Autodesk Inventor part; units mm, degrees
(part 2 of 10)
  spline S9 degree 5 poles (-7.9935, -0.3229) (-7.988, -0.3264) (-7.9807, -0.331) (-7.9716, -0.3367) (-7.9607, -0.3435) (-7.948, -0.3514) (-7.9389, -0.357) (-7.9299, -0.3625) (-7.9208, -0.368) (-7.9118, -0.3735) (-7.9028, -0.3789) (-7.8937, -0.3843) (-7.8847, -0.3897) (-7.8757, -0.3951) (-7.8667, -0.4004) (-7.8578, -0.4056) (-7.8488, -0.4109) (-7.8398, -0.4161) (-7.8309, -0.4212) (-7.822, -0.4263) (-7.813, -0.4314) (-7.8041, -0.4365) (-7.7952, -0.4415) (-7.7863, -0.4465) (-7.7775, -0.4514) (-7.7686, -0.4563) (-7.7598, -0.4612) (-7.7509, -0.4661) (-7.7421, -0.4709) (-7.7333, -0.4756) (-7.7227, -0.4813) (-7.7122, -0.487) (-7.7017, -0.4925) (-7.6912, -0.4981) (-7.6772, -0.5054) (-7.665, -0.5117) (-7.6529, -0.5179) (-7.6408, -0.5241) (-7.6252, -0.5319) (-7.6131, -0.538) (-7.6011, -0.5439) (-7.5891, -0.5498) (-7.5737, -0.5573) (-7.5618, -0.563) (-7.5499, -0.5687) (-7.5364, -0.5751) (-7.5229, -0.5814) (-7.5128, -0.586) (-7.501, -0.5914) (-7.4893, -0.5967) (-7.4793, -0.6013) (-7.4677, -0.6065) (-7.4561, -0.6116) (-7.4462, -0.6159) (-7.4346, -0.6209) (-7.4231, -0.6259) (-7.4133, -0.6301) (-7.4019, -0.6349) (-7.3905, -0.6397) (-7.3808, -0.6437) (-7.3695, -0.6483) (-7.3582, -0.6529) (-7.3486, -0.6568) (-7.3374, -0.6612) (-7.3263, -0.6656) (-7.3168, -0.6693) (-7.3057, -0.6736) (-7.2947, -0.6778) (-7.2853, -0.6814) (-7.2744, -0.6855) (-7.2635, -0.6895) (-7.2542, -0.6929) (-7.2434, -0.6968) (-7.2327, -0.7006) (-7.2235, -0.7039) (-7.2129, -0.7076) (-7.2023, -0.7113) (-7.1932, -0.7144) (-7.1827, -0.718) (-7.1723, -0.7215) (-7.1634, -0.7244) (-7.153, -0.7278) (-7.1427, -0.7311) (-7.134, -0.7339) (-7.1238, -0.7371) (-7.1136, -0.7403) (-7.105, -0.7429) (-7.095, -0.746) (-7.085, -0.749) (-7.0765, -0.7515) (-7.0666, -0.7544) (-7.0568, -0.7572) (-7.0485, -0.7595) (-7.0388, -0.7623) (-7.0292, -0.7649) (-7.021, -0.7671) (-7.0114, -0.7697) (-7.002, -0.7722) (-6.9939, -0.7743) (-6.9846, -0.7767) (-6.9754, -0.779) (-6.9675, -0.781) (-6.9583, -0.7832) (-6.9493, -0.7854) (-6.9416, -0.7872) (-6.9326, -0.7893) (-6.9237, -0.7913) (-6.9162, -0.793) (-6.9075, -0.7949) (-6.8988, -0.7968) (-6.8914, -0.7984) (-6.8829, -0.8002) (-6.8744, -0.8019) (-6.8673, -0.8033) (-6.8589, -0.805) (-6.8507, -0.8066) (-6.8437, -0.8079) (-6.8356, -0.8094) (-6.8276, -0.8108) (-6.8208, -0.812) (-6.8129, -0.8134) (-6.8052, -0.8147) (-6.7986, -0.8158) (-6.7909, -0.8171) (-6.7834, -0.8182) (-6.777, -0.8192) (-6.7696, -0.8203) (-6.7623, -0.8214) (-6.7561, -0.8223) (-6.749, -0.8232) (-6.7419, -0.8242) (-6.736, -0.8249) (-6.7291, -0.8258) (-6.7223, -0.8266) (-6.7166, -0.8273) (-6.7099, -0.828) (-6.7034, -0.8287) (-6.6979, -0.8293) (-6.6916, -0.83) (-6.6853, -0.8306) (-6.6801, -0.8311) (-6.674, -0.8316) (-6.668, -0.8321) (-6.663, -0.8325) (-6.6573, -0.8329) (-6.6516, -0.8333) (-6.6468, -0.8337) (-6.6406, -0.8341) (-6.6345, -0.8344) (-6.6292, -0.8347) (-6.6241, -0.8349) (-6.617, -0.8353) (-6.6115, -0.8355) (-6.6061, -0.8356) (-6.6009, -0.8358) (-6.5959, -0.8359) (-6.5922, -0.836) (-6.5885, -0.836) (-6.585, -0.836) (-6.5816, -0.8361) (-6.5782, -0.8361) (-6.5755, -0.8361) (-6.5729, -0.8361) (-6.5703, -0.836) (-6.5678, -0.836) (-6.5653, -0.836) (-6.5629, -0.8359) (-6.5606, -0.8359) (-6.5583, -0.8358) (-6.5561, -0.8358) (-6.554, -0.8357) (-6.5519, -0.8356) (-6.55, -0.8356) (-6.548, -0.8355) (-6.5462, -0.8354) (-6.5444, -0.8353) (-6.5427, -0.8352) (-6.5411, -0.8351) (-6.5395, -0.835) (-6.5381, -0.8349) (-6.5366, -0.8349) (-6.5353, -0.8348) (-6.5341, -0.8347) (-6.5329, -0.8346) (-6.5318, -0.8345) (-6.5307, -0.8344) (-6.5298, -0.8343) (-6.5289, -0.8343) (-6.5281, -0.8342) (-6.5274, -0.8341) (-6.5267, -0.834) (-6.5262, -0.834) (-6.5258, -0.8339) (-6.5256, -0.8339) (-6.5254, -0.8339) knots -1 -1 -1 -1 -1 -1 -0.9875 -0.983333 -0.979167 -0.975 -0.970833 -0.966667 -0.9625 -0.958333 -0.954167 -0.95 -0.945833 -0.941667 -0.9375 -0.933333 -0.929167 -0.925 -0.920833 -0.916667 -0.9125 -0.908333 -0.904167 -0.9 -0.895833 -0.891667 -0.8875 -0.883333 -0.879167 -0.875 -0.870833 -0.8625 -0.858333 -0.854167 -0.85 -0.8375 -0.833333 -0.829167 -0.825 -0.8125 -0.808333 -0.804167 -0.8 -0.7875 -0.783333 -0.779167 -0.770833 -0.766667 -0.7625 -0.754167 -0.75 -0.745833 -0.7375 -0.733333 -0.729167 -0.720833 -0.716667 -0.7125 -0.704167 -0.7 -0.695833 -0.6875 -0.683333 -0.679167 -0.670833 -0.666667 -0.6625 -0.654167 -0.65 -0.645833 -0.6375 -0.633333 -0.629167 -0.620833 -0.616667 -0.6125 -0.604167 -0.6 -0.595833 -0.5875 -0.583333 -0.579167 -0.570833 -0.566667 -0.5625 -0.554167 -0.55 -0.545833 -0.5375 -0.533333 -0.529167 -0.520833 -0.516667 -0.5125 -0.504167 -0.5 -0.495833 -0.4875 -0.483333 -0.479167 -0.470833 -0.466667 -0.4625 -0.454167 -0.45 -0.445833 -0.4375 -0.433333 -0.429167 -0.420833 -0.416667 -0.4125 -0.404167 -0.4 -0.395833 -0.3875 -0.383333 -0.379167 -0.370833 -0.366667 -0.3625 -0.354167 -0.35 -0.345833 -0.3375 -0.333333 -0.329167 -0.320833 -0.316667 -0.3125 -0.304167 -0.3 -0.295833 -0.2875 -0.283333 -0.279167 -0.270833 -0.266667 -0.2625 -0.254167 -0.25 -0.245833 -0.2375 -0.233333 -0.229167 -0.220833 -0.216667 -0.2125 -0.2 -0.195833 -0.191667 -0.1875 -0.170833 -0.166667 -0.1625 -0.158333 -0.154167 -0.145833 -0.141667 -0.1375 -0.133333 -0.129167 -0.125 -0.120833 -0.116667 -0.1125 -0.108333 -0.104167 -0.1 -0.095833 -0.091667 -0.0875 -0.083333 -0.079167 -0.075 -0.070833 -0.066667 -0.0625 -0.058333 -0.054167 -0.05 -0.045833 -0.041667 -0.0375 -0.033333 -0.029167 -0.025 -0.020833 -0.016667 -0.0125 -0.008333 0 0 0 0 0 0
  line L19 (-6.2404, 2.0798) -> (-5.455, 1.818)
  spline S10 degree 5 poles (-1.4639, -7.8649) (-1.4593, -7.8604) (-1.4532, -7.8543) (-1.4456, -7.8467) (-1.4365, -7.8376) (-1.426, -7.8269) (-1.4186, -7.8193) (-1.4111, -7.8117) (-1.4038, -7.8041) (-1.3964, -7.7965) (-1.3891, -7.7889) (-1.3818, -7.7813) (-1.3746, -7.7738) (-1.3674, -7.7662) (-1.3602, -7.7586) (-1.3531, -7.751) (-1.346, -7.7434) (-1.3389, -7.7359) (-1.3319, -7.7283) (-1.3249, -7.7207) (-1.318, -7.7132) (-1.311, -7.7056) (-1.3042, -7.698) (-1.2973, -7.6905) (-1.2905, -7.6829) (-1.2838, -7.6754) (-1.2771, -7.6678) (-1.2704, -7.6603) (-1.2637, -7.6528) (-1.2571, -7.6452) (-1.2492, -7.6362) (-1.2414, -7.6272) (-1.2336, -7.6182) (-1.2259, -7.6092) (-1.2156, -7.5972) (-1.2068, -7.5867) (-1.198, -7.5763) (-1.1893, -7.5658) (-1.1782, -7.5524) (-1.1696, -7.542) (-1.1611, -7.5316) (-1.1527, -7.5212) (-1.142, -7.5079) (-1.1338, -7.4975) (-1.1256, -7.4872) (-1.1163, -7.4754) (-1.1072, -7.4636) (-1.1004, -7.4548) (-1.0925, -7.4446) (-1.0847, -7.4343) (-1.0781, -7.4256) (-1.0705, -7.4154) (-1.0629, -7.4052) (-1.0564, -7.3965) (-1.049, -7.3864) (-1.0416, -7.3763) (-1.0353, -7.3676) (-1.0281, -7.3576) (-1.0209, -7.3475) (-1.0148, -7.339) (-1.0078, -7.329) (-1.0008, -7.319) (-0.9949, -7.3105) (-0.9881, -7.3006) (-0.9813, -7.2907) (-0.9756, -7.2823) (-0.969, -7.2724) (-0.9624, -7.2626) (-0.9569, -7.2543) (-0.9504, -7.2445) (-0.9441, -7.2348) (-0.9387, -7.2265) (-0.9325, -7.2169) (-0.9263, -7.2073) (-0.9211, -7.199) (-0.9151, -7.1895) (-0.9092, -7.18) (-0.9042, -7.1719) (-0.8984, -7.1624) (-0.8926, -7.153) (-0.8878, -7.145) (-0.8822, -7.1356) (-0.8766, -7.1263) (-0.8719, -7.1184) (-0.8665, -7.1092) (-0.8612, -7.1) (-0.8567, -7.0922) (-0.8515, -7.0831) (-0.8464, -7.074) (-0.842, -7.0663) (-0.837, -7.0573) (-0.8321, -7.0484) (-0.8279, -7.0408) (-0.8231, -7.0319) (-0.8184, -7.0231) (-0.8144, -7.0156) (-0.8098, -7.0069) (-0.8053, -6.9983) (-0.8014, -6.9909) (-0.797, -6.9823) (-0.7927, -6.9738) (-0.789, -6.9666) (-0.7842, -6.957) (-0.7795, -6.9474) (-0.7754, -6.9391) (-0.7715, -6.9309) (-0.7664, -6.9204) (-0.7626, -6.9123) (-0.7588, -6.9043) (-0.7551, -6.8963) (-0.7499, -6.885) (-0.7459, -6.876) (-0.7419, -6.8672) (-0.7381, -6.8584) (-0.7334, -6.8476) (-0.7301, -6.84) (-0.727, -6.8326) (-0.7239, -6.8252) (-0.7196, -6.8148) (-0.7162, -6.8065) (-0.7129, -6.7984) (-0.7097, -6.7903) (-0.7059, -6.7804) (-0.7032, -6.7736) (-0.7006, -6.7668) (-0.6981, -6.7601) (-0.695, -6.7516) (-0.6926, -6.745) (-0.6903, -6.7386) (-0.6877, -6.7313) (-0.6852, -6.7242) (-0.6834, -6.7189) (-0.6813, -6.7128) (-0.6793, -6.7068) (-0.6776, -6.7017) (-0.6757, -6.6958) (-0.6738, -6.6901) (-0.6723, -6.6852) (-0.6705, -6.6796) (-0.6689, -6.6741) (-0.6674, -6.6695) (-0.6658, -6.6642) (-0.6643, -6.6589) (-0.663, -6.6545) (-0.6614, -6.6488) (-0.6598, -6.6432) (-0.6585, -6.6383) (-0.6572, -6.6336) (-0.656, -6.6291) (-0.6548, -6.6245) (-0.6537, -6.6201) (-0.6526, -6.6159) (-0.6516, -6.6117) (-0.6506, -6.6077) (-0.65, -6.6048) (-0.6493, -6.6021) (-0.6487, -6.5994) (-0.6481, -6.5967) (-0.6475, -6.5941) (-0.6469, -6.5916) (-0.6464, -6.5891) (-0.6459, -6.5867) (-0.6454, -6.5844) (-0.6449, -6.5821) (-0.6445, -6.5799) (-0.6441, -6.5777) (-0.6437, -6.5756) (-0.6433, -6.5736) (-0.6429, -6.5717) (-0.6425, -6.5698) (-0.6422, -6.568) (-0.6419, -6.5662) (-0.6416, -6.5645) (-0.6413, -6.5629) (-0.6411, -6.5614) (-0.6408, -6.5599) (-0.6406, -6.5585) (-0.6404, -6.5572) (-0.6402, -6.556) (-0.64, -6.5548) (-0.6399, -6.5537) (-0.6397, -6.5527) (-0.6396, -6.5517) (-0.6395, -6.5509) (-0.6394, -6.5501) (-0.6393, -6.5494) (-0.6392, -6.5486) (-0.6391, -6.5481) (-0.6391, -6.5478) (-0.6391, -6.5475) (-0.6391, -6.5474) knots -1 -1 -1 -1 -1 -1 -0.9875 -0.983333 -0.979167 -0.975 -0.970833 -0.966667 -0.9625 -0.958333 -0.954167 -0.95 -0.945833 -0.941667 -0.9375 -0.933333 -0.929167 -0.925 -0.920833 -0.916667 -0.9125 -0.908333 -0.904167 -0.9 -0.895833 -0.891667 -0.8875 -0.883333 -0.879167 -0.875 -0.870833 -0.8625 -0.858333 -0.854167 -0.85 -0.8375 -0.833333 -0.829167 -0.825 -0.8125 -0.808333 -0.804167 -0.8 -0.7875 -0.783333 -0.779167 -0.770833 -0.766667 -0.7625 -0.754167 -0.75 -0.745833 -0.7375 -0.733333 -0.729167 -0.720833 -0.716667 -0.7125 -0.704167 -0.7 -0.695833 -0.6875 -0.683333 -0.679167 -0.670833 -0.666667 -0.6625 -0.654167 -0.65 -0.645833 -0.6375 -0.633333 -0.629167 -0.620833 -0.616667 -0.6125 -0.604167 -0.6 -0.595833 -0.5875 -0.583333 -0.579167 -0.570833 -0.566667 -0.5625 -0.554167 -0.55 -0.545833 -0.5375 -0.533333 -0.529167 -0.520833 -0.516667 -0.5125 -0.504167 -0.5 -0.495833 -0.4875 -0.483333 -0.479167 -0.470833 -0.466667 -0.4625 -0.45 -0.445833 -0.441667 -0.4375 -0.425 -0.420833 -0.416667 -0.4125 -0.395833 -0.391667 -0.3875 -0.383333 -0.370833 -0.366667 -0.3625 -0.358333 -0.341667 -0.3375 -0.333333 -0.329167 -0.316667 -0.3125 -0.308333 -0.304167 -0.291667 -0.2875 -0.283333 -0.275 -0.270833 -0.266667 -0.258333 -0.254167 -0.25 -0.241667 -0.2375 -0.233333 -0.225 -0.220833 -0.216667 -0.208333 -0.204167 -0.2 -0.1875 -0.183333 -0.179167 -0.175 -0.170833 -0.158333 -0.154167 -0.15 -0.145833 -0.141667 -0.1375 -0.133333 -0.129167 -0.125 -0.120833 -0.116667 -0.1125 -0.108333 -0.104167 -0.1 -0.095833 -0.091667 -0.0875 -0.083333 -0.079167 -0.075 -0.070833 -0.066667 -0.0625 -0.058333 -0.054167 -0.05 -0.045833 -0.041667 -0.0375 -0.033333 -0.029167 -0.025 -0.020833 -0.016667 -0.0125 -0.008333 0 0 0 0 0 0
  line L20 (-1.9798, -5.3984) -> (-2.2648, -6.1757)
  line L21 (-2.2648, -6.1757) -> (-2.265, -6.1763)
  arc A11 (-2.9863, -4.9137) -> (-1.9798, -5.3984) centre (0, 0) ccw
  spline S11 degree 5 poles (-2.265, -6.1763) (-2.2651, -6.1763) (-2.2651, -6.1765) (-2.2652, -6.1767) (-2.2653, -6.177) (-2.2655, -6.1776) (-2.2657, -6.1782) (-2.2659, -6.1788) (-2.2662, -6.1796) (-2.2664, -6.1804) (-2.2667, -6.1813) (-2.267, -6.1823) (-2.2674, -6.1834) (-2.2677, -6.1845) (-2.2681, -6.1857) (-2.2685, -6.187) (-2.2689, -6.1883) (-2.2693, -6.1898) (-2.2697, -6.1913) (-2.2702, -6.1928) (-2.2706, -6.1945) (-2.2711, -6.1962) (-2.2716, -6.198) (-2.2721, -6.1998) (-2.2726, -6.2017) (-2.2732, -6.2037) (-2.2737, -6.2058) (-2.2742, -6.2079) (-2.2748, -6.2101) (-2.2754, -6.2123) (-2.2759, -6.2147) (-2.2765, -6.2171) (-2.2771, -6.2195) (-2.2777, -6.222) (-2.2783, -6.2246) (-2.279, -6.2278) (-2.2798, -6.2311) (-2.2805, -6.2344) (-2.2815, -6.2391) (-2.2828, -6.2451) (-2.2839, -6.2507) (-2.2851, -6.2565) (-2.2862, -6.2625) (-2.2875, -6.2694) (-2.2885, -6.2751) (-2.2895, -6.281) (-2.2906, -6.287) (-2.2918, -6.2947) (-2.2927, -6.3002) (-2.2935, -6.3058) (-2.2944, -6.3115) (-2.2956, -6.3199) (-2.2966, -6.3268) (-2.2975, -6.3338) (-2.2984, -6.3409) (-2.2995, -6.35) (-2.3003, -6.3565) (-2.301, -6.3631) (-2.3017, -6.3698) (-2.3027, -6.3786) (-2.3033, -6.3855) (-2.304, -6.3925) (-2.3047, -6.4007) (-2.3055, -6.4089) (-2.306, -6.4152) (-2.3065, -6.4216) (-2.3072, -6.4312) (-2.3078, -6.4399) (-2.3083, -6.4488) (-2.3089, -6.4577) (-2.3095, -6.4691) (-2.3099, -6.4771) (-2.3102, -6.4853) (-2.3106, -6.4935) (-2.3109, -6.5042) (-2.3112, -6.5127) (-2.3114, -6.5212) (-2.3116, -6.5298) (-2.3119, -6.5422) (-2.312, -6.5523) (-2.3121, -6.5625) (-2.3121, -6.5728) (-2.3121, -6.5858) (-2.3121, -6.595) (-2.312, -6.6043) (-2.3119, -6.6136) (-2.3117, -6.6258) (-2.3115, -6.6353) (-2.3112, -6.6449) (-2.3109, -6.656) (-2.3105, -6.6672) (-2.3102, -6.6756) (-2.3097, -6.6856) (-2.3093, -6.6956) (-2.3089, -6.7042) (-2.3083, -6.7143) (-2.3077, -6.7245) (-2.3072, -6.7333) (-2.3065, -6.7437) (-2.3058, -6.7541) (-2.3052, -6.763) (-2.3044, -6.7736) (-2.3036, -6.7842) (-2.3028, -6.7933) (-2.3019, -6.804) (-2.301, -6.8148) (-2.3001, -6.8241) (-2.299, -6.8351) (-2.2979, -6.846) (-2.297, -6.8555) (-2.2958, -6.8666) (-2.2945, -6.8778) (-2.2934, -6.8874) (-2.2921, -6.8987) (-2.2907, -6.91) (-2.2895, -6.9198) (-2.288, -6.9312) (-2.2865, -6.9428) (-2.2852, -6.9527) (-2.2836, -6.9643) (-2.2819, -6.976) (-2.2804, -6.9861) (-2.2787, -6.9979) (-2.2768, -7.0097) (-2.2752, -7.0199) (-2.2733, -7.0319) (-2.2714, -7.0439) (-2.2696, -7.0542) (-2.2676, -7.0663) (-2.2654, -7.0785) (-2.2636, -7.089) (-2.2614, -7.1012) (-2.2591, -7.1136) (-2.2571, -7.1242) (-2.2547, -7.1366) (-2.2523, -7.1491) (-2.2501, -7.1598) (-2.2476, -7.1724) (-2.245, -7.185) (-2.2427, -7.1958) (-2.24, -7.2085) (-2.2372, -7.2213) (-2.2348, -7.2323) (-2.2324, -7.2433) (-2.2295, -7.2562) (-2.2269, -7.2672) (-2.2243, -7.2784) (-2.2212, -7.2914) (-2.2177, -7.3063) (-2.2145, -7.3194) (-2.2112, -7.3326) (-2.2074, -7.3476) (-2.2035, -7.3628) (-2.2001, -7.3761) (-2.196, -7.3913) (-2.1919, -7.4066) (-2.1883, -7.4201) (-2.1851, -7.4316) (-2.1818, -7.4432) (-2.1791, -7.4529) (-2.1764, -7.4626) (-2.1736, -7.4723) (-2.1708, -7.482) (-2.1679, -7.4918) (-2.165, -7.5015) (-2.1621, -7.5113) (-2.1592, -7.5211) (-2.1562, -7.531) (-2.1532, -7.5408) (-2.1501, -7.5507) (-2.1471, -7.5606) (-2.144, -7.5705) (-2.1408, -7.5804) (-2.1377, -7.5904) (-2.1345, -7.6003) (-2.1312, -7.6103) (-2.128, -7.6203) (-2.1247, -7.6303) (-2.1213, -7.6403) (-2.118, -7.6504) (-2.1146, -7.6605) (-2.1091, -7.6766) (-2.1042, -7.6907) (-2.1, -7.7029) (-2.0964, -7.7131) (-2.0935, -7.7212) knots 0 0 0 0 0 0 0.004167 0.008333 0.0125 0.016667 0.020833 0.025 0.029167 0.033333 0.0375 0.041667 0.045833 0.05 0.054167 0.058333 0.0625 0.066667 0.070833 0.075 0.079167 0.083333 0.0875 0.091667 0.095833 0.1 0.104167 0.108333 0.1125 0.116667 0.120833 0.125 0.129167 0.133333 0.1375 0.141667 0.15 0.154167 0.158333 0.170833 0.183333 0.1875 0.191667 0.195833 0.2125 0.216667 0.220833 0.225 0.2375 0.241667 0.245833 0.25 0.266667 0.270833 0.275 0.279167 0.291667 0.295833 0.3 0.304167 0.316667 0.320833 0.325 0.333333 0.3375 0.341667 0.345833 0.3625 0.366667 0.370833 0.375 0.3875 0.391667 0.395833 0.4 0.4125 0.416667 0.420833 0.425 0.441667 0.445833 0.45 0.454167 0.466667 0.470833 0.475 0.479167 0.491667 0.495833 0.5 0.508333 0.5125 0.516667 0.525 0.529167 0.533333 0.541667 0.545833 0.55 0.558333 0.5625 0.566667 0.575 0.579167 0.583333 0.591667 0.595833 0.6 0.608333 0.6125 0.616667 0.625 0.629167 0.633333 0.641667 0.645833 0.65 0.658333 0.6625 0.666667 0.675 0.679167 0.683333 0.691667 0.695833 0.7 0.708333 0.7125 0.716667 0.725 0.729167 0.733333 0.741667 0.745833 0.75 0.758333 0.7625 0.766667 0.775 0.779167 0.783333 0.791667 0.795833 0.8 0.804167 0.8125 0.816667 0.820833 0.829167 0.8375 0.841667 0.845833 0.854167 0.8625 0.866667 0.875 0.879167 0.883333 0.8875 0.891667 0.895833 0.9 0.904167 0.908333 0.9125 0.916667 0.920833 0.925 0.929167 0.933333 0.9375 0.941667 0.945833 0.95 0.954167 0.958333 0.9625 0.966667 0.970833 0.975 0.979167 0.983333 1 1 1 1 1 1
  arc A12 (-2.0935, -7.7212) -> (-1.4639, -7.8649) centre (0, 0) ccw
  line L22 (-2.2648, 6.1757) -> (-1.9798, 5.3984)
  arc A13 (-1.9798, 5.3984) -> (-2.9863, 4.9137) centre (0, 0) ccw
  line L23 (-3.4162, 5.6212) -> (-3.4166, 5.6217)
  line L24 (-2.9863, 4.9137) -> (-3.4162, 5.6212)
  spline S12 degree 5 poles (-3.4166, 5.6217) (-3.4166, 5.6218) (-3.4167, 5.6219) (-3.4168, 5.6221) (-3.417, 5.6224) (-3.4173, 5.6229) (-3.4176, 5.6234) (-3.418, 5.624) (-3.4185, 5.6247) (-3.419, 5.6254) (-3.4195, 5.6262) (-3.4201, 5.627) (-3.4207, 5.628) (-3.4213, 5.6289) (-3.4221, 5.63) (-3.4228, 5.6311) (-3.4236, 5.6322) (-3.4245, 5.6335) (-3.4254, 5.6347) (-3.4263, 5.6361) (-3.4273, 5.6374) (-3.4283, 5.6389) (-3.4294, 5.6404) (-3.4306, 5.6419) (-3.4317, 5.6435) (-3.433, 5.6452) (-3.4342, 5.6469) (-3.4356, 5.6486) (-3.4369, 5.6504) (-3.4383, 5.6523) (-3.4398, 5.6542) (-3.4413, 5.6561) (-3.4429, 5.6581) (-3.4445, 5.6602) (-3.4464, 5.6627) (-3.4485, 5.6652) (-3.4506, 5.6678) (-3.4542, 5.6723) (-3.4581, 5.677) (-3.4621, 5.6819) (-3.4664, 5.6869) (-3.4708, 5.6921) (-3.474, 5.6958) (-3.4773, 5.6995) (-3.4802, 5.7028) (-3.4837, 5.7067) (-3.4872, 5.7107) (-3.4903, 5.7141) (-3.494, 5.7182) (-3.4979, 5.7224) (-3.5012, 5.726) (-3.5052, 5.7302) (-3.5092, 5.7346) (-3.5128, 5.7383) (-3.517, 5.7427) (-3.5214, 5.7472) (-3.5251, 5.7511) (-3.5296, 5.7557) (-3.5342, 5.7603) (-3.5382, 5.7643) (-3.5429, 5.7691) (-3.5478, 5.7738) (-3.552, 5.778) (-3.557, 5.7828) (-3.5621, 5.7877) (-3.5665, 5.792) (-3.5718, 5.7969) (-3.5771, 5.802) (-3.5818, 5.8063) (-3.5873, 5.8114) (-3.5929, 5.8166) (-3.5977, 5.821) (-3.6035, 5.8262) (-3.6093, 5.8315) (-3.6144, 5.836) (-3.6204, 5.8413) (-3.6265, 5.8466) (-3.6318, 5.8513) (-3.638, 5.8567) (-3.6444, 5.8621) (-3.6499, 5.8668) (-3.6564, 5.8723) (-3.663, 5.8778) (-3.6687, 5.8825) (-3.6754, 5.8881) (-3.6823, 5.8937) (-3.6882, 5.8985) (-3.6952, 5.9041) (-3.7023, 5.9098) (-3.7084, 5.9147) (-3.7156, 5.9204) (-3.723, 5.9261) (-3.7293, 5.931) (-3.7368, 5.9368) (-3.7444, 5.9426) (-3.7509, 5.9475) (-3.7586, 5.9533) (-3.7664, 5.9592) (-3.7732, 5.9642) (-3.7811, 5.97) (-3.7892, 5.9759) (-3.7961, 5.9809) (-3.8043, 5.9868) (-3.8126, 5.9927) (-3.8198, 5.9978) (-3.8282, 6.0037) (-3.8367, 6.0096) (-3.8441, 6.0147) (-3.8528, 6.0207) (-3.8615, 6.0266) (-3.8691, 6.0317) (-3.878, 6.0377) (-3.887, 6.0437) (-3.8947, 6.0488) (-3.9039, 6.0548) (-3.9131, 6.0608) (-3.921, 6.0659) (-3.9304, 6.0719) (-3.9398, 6.0779) (-3.948, 6.083) (-3.9576, 6.089) (-3.9673, 6.095) (-3.9756, 6.1002) (-3.984, 6.1053) (-3.9967, 6.113) (-4.0081, 6.1198) (-4.0197, 6.1267) (-4.0313, 6.1335) (-4.046, 6.1421) (-4.0563, 6.148) (-4.0668, 6.154) (-4.0788, 6.1608) (-4.091, 6.1676) (-4.1001, 6.1727) (-4.1109, 6.1786) (-4.1217, 6.1846) (-4.1311, 6.1896) (-4.142, 6.1956) (-4.1531, 6.2015) (-4.1626, 6.2065) (-4.1738, 6.2124) (-4.1851, 6.2183) (-4.1948, 6.2233) (-4.2062, 6.2291) (-4.2177, 6.235) (-4.2276, 6.24) (-4.2392, 6.2458) (-4.2509, 6.2516) (-4.261, 6.2565) (-4.2712, 6.2615) (-4.283, 6.2672) (-4.2933, 6.2721) (-4.3036, 6.277) (-4.3157, 6.2827) (-4.3279, 6.2884) (-4.3383, 6.2933) (-4.3506, 6.2989) (-4.363, 6.3046) (-4.3737, 6.3094) (-4.3844, 6.3142) (-4.3987, 6.3206) (-4.4114, 6.3261) (-4.4241, 6.3317) (-4.4369, 6.3372) (-4.4498, 6.3427) (-4.459, 6.3466) (-4.4682, 6.3505) (-4.4775, 6.3544) (-4.4869, 6.3583) (-4.4962, 6.3621) (-4.5056, 6.366) (-4.5151, 6.3698) (-4.5245, 6.3737) (-4.534, 6.3775) (-4.5436, 6.3813) (-4.5532, 6.3851) (-4.5628, 6.3888) (-4.5724, 6.3926) (-4.5821, 6.3963) (-4.5918, 6.4001) (-4.6016, 6.4038) (-4.6114, 6.4075) (-4.6212, 6.4112) (-4.631, 6.4149) (-4.6409, 6.4186) (-4.6508, 6.4222) (-4.6608, 6.4258) (-4.6708, 6.4295) (-4.6868, 6.4352) (-4.7009, 6.4403) (-4.7131, 6.4445) (-4.7232, 6.4481) (-4.7314, 6.4509) knots 0 0 0 0 0 0 0.004167 0.008333 0.0125 0.016667 0.020833 0.025 0.029167 0.033333 0.0375 0.041667 0.045833 0.05 0.054167 0.058333 0.0625 0.066667 0.070833 0.075 0.079167 0.083333 0.0875 0.091667 0.095833 0.1 0.104167 0.108333 0.1125 0.116667 0.120833 0.125 0.129167 0.133333 0.1375 0.145833 0.15 0.154167 0.175 0.179167 0.1875 0.191667 0.195833 0.204167 0.208333 0.2125 0.220833 0.225 0.229167 0.2375 0.241667 0.245833 0.254167 0.258333 0.2625 0.270833 0.275 0.279167 0.2875 0.291667 0.295833 0.304167 0.308333 0.3125 0.320833 0.325 0.329167 0.3375 0.341667 0.345833 0.354167 0.358333 0.3625 0.370833 0.375 0.379167 0.3875 0.391667 0.395833 0.404167 0.408333 0.4125 0.420833 0.425 0.429167 0.4375 0.441667 0.445833 0.454167 0.458333 0.4625 0.470833 0.475 0.479167 0.4875 0.491667 0.495833 0.504167 0.508333 0.5125 0.520833 0.525 0.529167 0.5375 0.541667 0.545833 0.554167 0.558333 0.5625 0.570833 0.575 0.579167 0.5875 0.591667 0.595833 0.604167 0.608333 0.6125 0.620833 0.625 0.629167 0.6375 0.641667 0.645833 0.65 0.666667 0.670833 0.675 0.679167 0.691667 0.695833 0.7 0.708333 0.7125 0.716667 0.725 0.729167 0.733333 0.741667 0.745833 0.75 0.758333 0.7625 0.766667 0.775 0.779167 0.783333 0.791667 0.795833 0.8 0.804167 0.8125 0.816667 0.820833 0.829167 0.833333 0.8375 0.845833 0.85 0.854167 0.858333 0.870833 0.875 0.879167 0.883333 0.8875 0.891667 0.895833 0.9 0.904167 0.908333 0.9125 0.916667 0.920833 0.925 0.929167 0.933333 0.9375 0.941667 0.945833 0.95 0.954167 0.958333 0.9625 0.966667 0.970833 0.975 0.979167 0.983333 1 1 1 1 1 1
  arc A14 (-4.7314, 6.4509) -> (-5.2363, 6.0482) centre (0, 0) ccw
  line L25 (-4.7205, 4.5819) -> (-4.72, 4.5814)
  spline S13 degree 5 poles (-5.2363, 6.0482) (-5.2356, 6.0418) (-5.2347, 6.0332) (-5.2335, 6.0225) (-5.232, 6.0098) (-5.2302, 5.9949) (-5.2289, 5.9844) (-5.2276, 5.9738) (-5.2263, 5.9633) (-5.2249, 5.9528) (-5.2236, 5.9424) (-5.2222, 5.9319) (-5.2207, 5.9215) (-5.2193, 5.9112) (-5.2178, 5.9008) (-5.2164, 5.8905) (-5.2149, 5.8803) (-5.2133, 5.87) (-5.2118, 5.8598) (-5.2102, 5.8496) (-5.2087, 5.8395) (-5.207, 5.8294) (-5.2054, 5.8193) (-5.2038, 5.8092) (-5.2021, 5.7992) (-5.2004, 5.7892) (-5.1987, 5.7793) (-5.197, 5.7693) (-5.1953, 5.7594) (-5.1935, 5.7496) (-5.1917, 5.7397) (-5.1892, 5.726) (-5.1866, 5.7124) (-5.1841, 5.6988) (-5.1814, 5.6853) (-5.178, 5.668) (-5.1741, 5.6489) (-5.1702, 5.6299) (-5.1661, 5.6111) (-5.162, 5.5925) (-5.1578, 5.5739) (-5.1549, 5.561) (-5.1519, 5.5482) (-5.1489, 5.5355) (-5.1445, 5.5173) (-5.141, 5.5029) (-5.1374, 5.4886) (-5.1338, 5.4744) (-5.1293, 5.4568) (-5.126, 5.4446) (-5.1228, 5.4324) (-5.1195, 5.4203) (-5.1152, 5.4048) (-5.1119, 5.3929) (-5.1085, 5.381) (-5.1051, 5.3692) (-5.1007, 5.3541) (-5.0972, 5.3425) (-5.0938, 5.3309) (-5.0903, 5.3194) (-5.0857, 5.3048) (-5.0822, 5.2935) (-5.0786, 5.2822) (-5.0745, 5.2695) (-5.0704, 5.2568) (-5.0673, 5.2474) (-5.0636, 5.2365) (-5.0599, 5.2256) (-5.0568, 5.2164) (-5.0531, 5.2057) (-5.0493, 5.195) (-5.0461, 5.186) (-5.0424, 5.1755) (-5.0386, 5.1651) (-5.0354, 5.1562) (-5.0316, 5.146) (-5.0278, 5.1358) (-5.0245, 5.1271) (-5.0206, 5.1171) (-5.0168, 5.1072) (-5.0135, 5.0987) (-5.0096, 5.0889) (-5.0058, 5.0792) (-5.0024, 5.0709) (-4.9985, 5.0614) (-4.9946, 5.0519) (-4.9913, 5.0438) (-4.9874, 5.0345) (-4.9834, 5.0253) (-4.9801, 5.0174) (-4.9761, 5.0083) (-4.9722, 4.9993) (-4.9688, 4.9917) (-4.9649, 4.9828) (-4.9609, 4.9741) (-4.9575, 4.9666) (-4.9536, 4.958) (-4.9496, 4.9495) (-4.9463, 4.9423) (-4.9423, 4.9339) (-4.9384, 4.9257) (-4.935, 4.9187) (-4.931, 4.9106) (-4.9271, 4.9026) (-4.9237, 4.8958) (-4.9198, 4.8879) (-4.9159, 4.8802) (-4.9125, 4.8736) (-4.9086, 4.866) (-4.9047, 4.8585) (-4.9014, 4.8522) (-4.8975, 4.8448) (-4.8936, 4.8376) (-4.8903, 4.8315) (-4.8865, 4.8244) (-4.8827, 4.8174) (-4.8794, 4.8115) (-4.8756, 4.8047) (-4.8718, 4.798) (-4.8686, 4.7924) (-4.8648, 4.7858) (-4.8611, 4.7794) (-4.8579, 4.774) (-4.8542, 4.7677) (-4.8505, 4.7615) (-4.8474, 4.7563) (-4.8437, 4.7503) (-4.8401, 4.7445) (-4.8371, 4.7395) (-4.8335, 4.7338) (-4.83, 4.7282) (-4.827, 4.7234) (-4.8235, 4.718) (-4.82, 4.7127) (-4.8171, 4.7082) (-4.8137, 4.7031) (-4.8104, 4.698) (-4.8075, 4.6938) (-4.8043, 4.6889) (-4.801, 4.6842) (-4.7983, 4.6802) (-4.7956, 4.6763) (-4.7915, 4.6705) (-4.788, 4.6655) (-4.7846, 4.6607) (-4.7812, 4.6561) (-4.7774, 4.651) (-4.775, 4.6476) (-4.7726, 4.6444) (-4.7702, 4.6413) (-4.7679, 4.6382) (-4.766, 4.6357) (-4.7637, 4.6327) (-4.7615, 4.6299) (-4.7593, 4.6271) (-4.7572, 4.6244) (-4.7551, 4.6218) (-4.7534, 4.6197) (-4.7518, 4.6176) (-4.7501, 4.6156) (-4.7485, 4.6136) (-4.747, 4.6117) (-4.7455, 4.6099) (-4.744, 4.6081) (-4.7425, 4.6064) (-4.7411, 4.6047) (-4.7397, 4.6031) (-4.7384, 4.6015) (-4.7371, 4.6) (-4.7358, 4.5986) (-4.7346, 4.5972) (-4.7335, 4.5958) (-4.7323, 4.5946) (-4.7312, 4.5933) (-4.7302, 4.5922) (-4.7292, 4.5911) (-4.7282, 4.59) (-4.7273, 4.589) (-4.7265, 4.5881) (-4.7257, 4.5872) (-4.7249, 4.5864) (-4.7242, 4.5857) (-4.7236, 4.585) (-4.723, 4.5844) (-4.7224, 4.5838) (-4.7219, 4.5833) (-4.7214, 4.5827) (-4.721, 4.5824) (-4.7208, 4.5821) (-4.7206, 4.582) (-4.7205, 4.5819) knots -1 -1 -1 -1 -1 -1 -0.9875 -0.983333 -0.979167 -0.975 -0.970833 -0.966667 -0.9625 -0.958333 -0.954167 -0.95 -0.945833 -0.941667 -0.9375 -0.933333 -0.929167 -0.925 -0.920833 -0.916667 -0.9125 -0.908333 -0.904167 -0.9 -0.895833 -0.891667 -0.8875 -0.883333 -0.879167 -0.875 -0.870833 -0.866667 -0.854167 -0.85 -0.845833 -0.841667 -0.829167 -0.8125 -0.808333 -0.804167 -0.8 -0.7875 -0.783333 -0.779167 -0.775 -0.758333 -0.754167 -0.75 -0.745833 -0.733333 -0.729167 -0.725 -0.720833 -0.708333 -0.704167 -0.7 -0.695833 -0.683333 -0.679167 -0.675 -0.670833 -0.658333 -0.654167 -0.65 -0.641667 -0.6375 -0.633333 -0.625 -0.620833 -0.616667 -0.608333 -0.604167 -0.6 -0.591667 -0.5875 -0.583333 -0.575 -0.570833 -0.566667 -0.558333 -0.554167 -0.55 -0.541667 -0.5375 -0.533333 -0.525 -0.520833 -0.516667 -0.508333 -0.504167 -0.5 -0.491667 -0.4875 -0.483333 -0.475 -0.470833 -0.466667 -0.458333 -0.454167 -0.45 -0.441667 -0.4375 -0.433333 -0.425 -0.420833 -0.416667 -0.408333 -0.404167 -0.4 -0.391667 -0.3875 -0.383333 -0.375 -0.370833 -0.366667 -0.358333 -0.354167 -0.35 -0.341667 -0.3375 -0.333333 -0.325 -0.320833 -0.316667 -0.308333 -0.304167 -0.3 -0.291667 -0.2875 -0.283333 -0.275 -0.270833 -0.266667 -0.258333 -0.254167 -0.25 -0.241667 -0.2375 -0.233333 -0.225 -0.220833 -0.216667 -0.2125 -0.195833 -0.191667 -0.1875 -0.183333 -0.175 -0.170833 -0.166667 -0.1625 -0.158333 -0.154167 -0.145833 -0.141667 -0.1375 -0.133333 -0.129167 -0.125 -0.120833 -0.116667 -0.1125 -0.108333 -0.104167 -0.1 -0.095833 -0.091667 -0.0875 -0.083333 -0.079167 -0.075 -0.070833 -0.066667 -0.0625 -0.058333 -0.054167 -0.05 -0.045833 -0.041667 -0.0375 -0.033333 -0.029167 -0.025 -0.020833 -0.016667 -0.0125 -0.008333 0 0 0 0 0 0
  line L26 (-4.72, 4.5814) -> (-4.126, 4.0048)
  line L27 (-6.241, 2.08) -> (-6.2404, 2.0798)
  spline S14 degree 5 poles (-7.342, 3.1773) (-7.3386, 3.1718) (-7.334, 3.1645) (-7.3283, 3.1554) (-7.3214, 3.1445) (-7.3134, 3.1319) (-7.3076, 3.123) (-7.3019, 3.114) (-7.2961, 3.1051) (-7.2903, 3.0963) (-7.2846, 3.0875) (-7.2788, 3.0787) (-7.273, 3.0699) (-7.2672, 3.0612) (-7.2614, 3.0525) (-7.2556, 3.0439) (-7.2498, 3.0353) (-7.244, 3.0267) (-7.2381, 3.0182) (-7.2323, 3.0097) (-7.2265, 3.0012) (-7.2207, 2.9928) (-7.2148, 2.9844) (-7.209, 2.9761) (-7.2031, 2.9678) (-7.1973, 2.9595) (-7.1914, 2.9513) (-7.1856, 2.9431) (-7.1797, 2.9349) (-7.1738, 2.9268) (-7.1668, 2.9171) (-7.1597, 2.9075) (-7.1527, 2.8979) (-7.1456, 2.8883) (-7.1362, 2.8757) (-7.128, 2.8647) (-7.1197, 2.8538) (-7.1115, 2.843) (-7.1021, 2.8307) (-7.095, 2.8216) (-7.0855, 2.8094) (-7.0761, 2.7974) (-7.0667, 2.7855) (-7.0572, 2.7737) (-7.0478, 2.762) (-7.0407, 2.7533) (-7.0325, 2.7431) (-7.0242, 2.7331) (-7.0172, 2.7246) (-7.0101, 2.7161) (-6.9995, 2.7034) (-6.9901, 2.6923) (-6.9807, 2.6813) (-6.9713, 2.6704) (-6.9596, 2.6569) (-6.9514, 2.6475) (-6.9432, 2.6382) (-6.935, 2.629) (-6.9233, 2.6159) (-6.914, 2.6056) (-6.9046, 2.5954) (-6.8953, 2.5853) (-6.8849, 2.5741) (-6.878, 2.5666) (-6.871, 2.5593) (-6.8618, 2.5495) (-6.8525, 2.5399) (-6.8445, 2.5315) (-6.8364, 2.5232) (-6.8261, 2.5127) (-6.8181, 2.5046) (-6.8102, 2.4965) (-6.8011, 2.4875) (-6.792, 2.4785) (-6.7852, 2.4718) (-6.7773, 2.4641) (-6.7694, 2.4565) (-6.7627, 2.45) (-6.7548, 2.4425) (-6.747, 2.4351) (-6.7403, 2.4288) (-6.7326, 2.4216) (-6.7248, 2.4144) (-6.7182, 2.4083) (-6.7105, 2.4013) (-6.7028, 2.3943) (-6.6963, 2.3884) (-6.6887, 2.3816) (-6.6811, 2.3749) (-6.6746, 2.3691) (-6.6671, 2.3625) (-6.6596, 2.356) (-6.6532, 2.3505) (-6.6457, 2.3441) (-6.6383, 2.3379) (-6.632, 2.3325) (-6.6247, 2.3264) (-6.6174, 2.3203) (-6.6111, 2.3152) (-6.6039, 2.3093) (-6.5967, 2.3034) (-6.5906, 2.2985) (-6.5834, 2.2928) (-6.5764, 2.2872) (-6.5703, 2.2824) (-6.5643, 2.2777) (-6.5554, 2.2708) (-6.5475, 2.2647) (-6.5396, 2.2587) (-6.5319, 2.2529) (-6.5222, 2.2457) (-6.5155, 2.2408) (-6.5089, 2.2359) (-6.5023, 2.2312) (-6.4939, 2.2251) (-6.4875, 2.2205) (-6.4811, 2.216) (-6.4747, 2.2116) (-6.4657, 2.2054) (-6.4586, 2.2005) (-6.4516, 2.1958) (-6.4447, 2.1911) (-6.437, 2.186) (-6.4319, 2.1827) (-6.4268, 2.1794) (-6.4202, 2.1751) (-6.4136, 2.1709) (-6.4079, 2.1673) (-6.4023, 2.1638) (-6.3944, 2.1589) (-6.3882, 2.1551) (-6.3821, 2.1514) (-6.3761, 2.1478) (-6.3687, 2.1435) (-6.3637, 2.1405) (-6.3587, 2.1376) (-6.3537, 2.1348) (-6.3482, 2.1317) (-6.3442, 2.1294) (-6.3395, 2.1268) (-6.3349, 2.1243) (-6.3304, 2.1219) (-6.326, 2.1195) (-6.3217, 2.1172) (-6.3175, 2.115) (-6.3133, 2.1128) (-6.3093, 2.1107) (-6.3059, 2.109) (-6.302, 2.1071) (-6.2988, 2.1054) (-6.2956, 2.1039) (-6.2926, 2.1024) (-6.2896, 2.1009) (-6.2871, 2.0997) (-6.2847, 2.0986) (-6.2824, 2.0975) (-6.2801, 2.0964) (-6.2778, 2.0954) (-6.2757, 2.0944) (-6.2736, 2.0934) (-6.2715, 2.0925) (-6.2695, 2.0916) (-6.2675, 2.0907) (-6.2657, 2.0899) (-6.2638, 2.0891) (-6.2621, 2.0884) (-6.2604, 2.0876) (-6.2587, 2.0869) (-6.2572, 2.0863) (-6.2557, 2.0856) (-6.2542, 2.0851) (-6.2529, 2.0845) (-6.2515, 2.084) (-6.2503, 2.0835) (-6.2491, 2.083) (-6.248, 2.0826) (-6.247, 2.0822) (-6.246, 2.0818) (-6.2451, 2.0815) (-6.2443, 2.0812) (-6.2436, 2.0809) (-6.2429, 2.0806) (-6.2422, 2.0804) (-6.2417, 2.0802) (-6.2414, 2.0801) (-6.2412, 2.08) (-6.241, 2.08) knots -1 -1 -1 -1 -1 -1 -0.9875 -0.983333 -0.979167 -0.975 -0.970833 -0.966667 -0.9625 -0.958333 -0.954167 -0.95 -0.945833 -0.941667 -0.9375 -0.933333 -0.929167 -0.925 -0.920833 -0.916667 -0.9125 -0.908333 -0.904167 -0.9 -0.895833 -0.891667 -0.8875 -0.883333 -0.879167 -0.875 -0.870833 -0.8625 -0.858333 -0.854167 -0.85 -0.8375 -0.833333 -0.829167 -0.825 -0.816667 -0.8125 -0.8 -0.795833 -0.791667 -0.783333 -0.779167 -0.775 -0.766667 -0.7625 -0.758333 -0.754167 -0.7375 -0.733333 -0.729167 -0.725 -0.7125 -0.708333 -0.704167 -0.7 -0.683333 -0.679167 -0.675 -0.670833 -0.6625 -0.658333 -0.654167 -0.641667 -0.6375 -0.633333 -0.629167 -0.616667 -0.6125 -0.608333 -0.6 -0.595833 -0.591667 -0.583333 -0.579167 -0.575 -0.566667 -0.5625 -0.558333 -0.55 -0.545833 -0.541667 -0.533333 -0.529167 -0.525 -0.516667 -0.5125 -0.508333 -0.5 -0.495833 -0.491667 -0.483333 -0.479167 -0.475 -0.466667 -0.4625 -0.458333 -0.45 -0.445833 -0.441667 -0.433333 -0.429167 -0.425 -0.420833 -0.404167 -0.4 -0.395833 -0.391667 -0.379167 -0.375 -0.370833 -0.366667 -0.354167 -0.35 -0.345833 -0.341667 -0.325 -0.320833 -0.316667 -0.3125 -0.304167 -0.3 -0.295833 -0.283333 -0.279167 -0.275 -0.270833 -0.254167 -0.25 -0.245833 -0.241667 -0.229167 -0.225 -0.220833 -0.216667 -0.208333 -0.204167 -0.195833 -0.191667 -0.1875 -0.179167 -0.175 -0.166667 -0.1625 -0.158333 -0.154167 -0.145833 -0.141667 -0.1375 -0.133333 -0.129167 -0.125 -0.120833 -0.116667 -0.1125 -0.108333 -0.104167 -0.1 -0.095833 -0.091667 -0.0875 -0.083333 -0.079167 -0.075 -0.070833 -0.066667 -0.0625 -0.058333 -0.054167 -0.05 -0.045833 -0.041667 -0.0375 -0.033333 -0.029167 -0.025 -0.020833 -0.016667 -0.0125 -0.008333 0 0 0 0 0 0
  arc A15 (-7.0618, 3.7592) -> (-7.342, 3.1773) centre (0, 0) ccw
  spline S15 degree 5 poles (-5.5174, 3.5826) (-5.5175, 3.5826) (-5.5176, 3.5827) (-5.5178, 3.5828) (-5.5181, 3.583) (-5.5186, 3.5833) (-5.5191, 3.5837) (-5.5197, 3.584) (-5.5204, 3.5844) (-5.5211, 3.5849) (-5.522, 3.5854) (-5.5228, 3.5859) (-5.5238, 3.5864) (-5.5248, 3.587) (-5.5259, 3.5877) (-5.5271, 3.5883) (-5.5283, 3.589) (-5.5296, 3.5897) (-5.531, 3.5905) (-5.5324, 3.5913) (-5.5339, 3.5921) (-5.5355, 3.593) (-5.5371, 3.5938) (-5.5388, 3.5947) (-5.5405, 3.5957) (-5.5424, 3.5966) (-5.5442, 3.5976) (-5.5462, 3.5986) (-5.5482, 3.5996) (-5.5503, 3.6007) (-5.5524, 3.6018) (-5.5546, 3.6029) (-5.5569, 3.604) (-5.5592, 3.6051) (-5.5616, 3.6063) (-5.5645, 3.6077) (-5.5676, 3.6092) (-5.5707, 3.6106) (-5.5749, 3.6126) (-5.5805, 3.6152) (-5.5857, 3.6176) (-5.5912, 3.62) (-5.5968, 3.6224) (-5.6032, 3.6252) (-5.6085, 3.6275) (-5.614, 3.6298) (-5.6196, 3.6321) (-5.6269, 3.635) (-5.632, 3.6371) (-5.6373, 3.6392) (-5.6435, 3.6416) (-5.6499, 3.6441) (-5.6547, 3.6459) (-5.6596, 3.6477) (-5.6671, 3.6505) (-5.6739, 3.653) (-5.6808, 3.6555) (-5.6879, 3.658) (-5.697, 3.6611) (-5.7035, 3.6633) (-5.71, 3.6656) (-5.7167, 3.6678) (-5.7254, 3.6706) (-5.7322, 3.6728) (-5.7392, 3.675) (-5.7463, 3.6772) (-5.7556, 3.6801) (-5.7628, 3.6823) (-5.7702, 3.6845) (-5.7788, 3.687) (-5.7875, 3.6895) (-5.7941, 3.6914) (-5.8019, 3.6935) (-5.8098, 3.6957) (-5.8166, 3.6976) (-5.8246, 3.6997) (-5.8328, 3.7019) (-5.8398, 3.7037) (-5.8481, 3.7058) (-5.8565, 3.7079) (-5.8638, 3.7097) (-5.8723, 3.7118) (-5.881, 3.7138) (-5.8885, 3.7156) (-5.8973, 3.7176) (-5.9062, 3.7196) (-5.9139, 3.7214) (-5.9229, 3.7233) (-5.9321, 3.7253) (-5.94, 3.727) (-5.9493, 3.7289) (-5.9586, 3.7308) (-5.9667, 3.7324) (-5.9763, 3.7343) (-5.9859, 3.7361) (-5.9942, 3.7377) (-6.004, 3.7395) (-6.0138, 3.7413) (-6.0223, 3.7428) (-6.0323, 3.7445) (-6.0424, 3.7462) (-6.0511, 3.7477) (-6.0613, 3.7493) (-6.0716, 3.751) (-6.0805, 3.7523) (-6.091, 3.7539) (-6.1015, 3.7555) (-6.1106, 3.7568) (-6.1212, 3.7582) (-6.132, 3.7597) (-6.1412, 3.7609) (-6.1521, 3.7623) (-6.1631, 3.7637) (-6.1725, 3.7649) (-6.1836, 3.7662) (-6.1947, 3.7675) (-6.2044, 3.7685) (-6.2157, 3.7697) (-6.227, 3.7709) (-6.2368, 3.7719) (-6.2483, 3.773) (-6.2599, 3.7741) (-6.2699, 3.775) (-6.2816, 3.776) (-6.2933, 3.777) (-6.3035, 3.7778) (-6.3153, 3.7787) (-6.3273, 3.7796) (-6.3376, 3.7803) (-6.3497, 3.7811) (-6.3618, 3.7818) (-6.3723, 3.7824) (-6.3846, 3.7831) (-6.3969, 3.7838) (-6.4075, 3.7843) (-6.42, 3.7848) (-6.4325, 3.7854) (-6.4433, 3.7858) (-6.4559, 3.7862) (-6.4686, 3.7866) (-6.4796, 3.7869) (-6.4924, 3.7872) (-6.5053, 3.7875) (-6.5164, 3.7877) (-6.5294, 3.7879) (-6.5424, 3.788) (-6.5536, 3.7881) (-6.5649, 3.7882) (-6.5781, 3.7882) (-6.5895, 3.7882) (-6.6009, 3.7881) (-6.6143, 3.788) (-6.6277, 3.7879) (-6.6393, 3.7877) (-6.6547, 3.7874) (-6.6703, 3.7871) (-6.6839, 3.7868) (-6.6996, 3.7863) (-6.7154, 3.7858) (-6.7272, 3.7853) (-6.7392, 3.7849) (-6.7511, 3.7843) (-6.7611, 3.7839) (-6.7711, 3.7834) (-6.7811, 3.7829) (-6.7912, 3.7824) (-6.8013, 3.7818) (-6.8114, 3.7812) (-6.8215, 3.7806) (-6.8317, 3.78) (-6.8419, 3.7793) (-6.8521, 3.7787) (-6.8624, 3.7779) (-6.8726, 3.7772) (-6.8829, 3.7764) (-6.8933, 3.7756) (-6.9036, 3.7748) (-6.914, 3.774) (-6.9244, 3.7731) (-6.9348, 3.7722) (-6.9452, 3.7713) (-6.9557, 3.7703) (-6.9662, 3.7693) (-6.9767, 3.7683) (-6.9873, 3.7673) (-6.9979, 3.7662) (-7.0148, 3.7644) (-7.0297, 3.7628) (-7.0425, 3.7614) (-7.0532, 3.7602) (-7.0618, 3.7592) knots 0 0 0 0 0 0 0.004167 0.008333 0.0125 0.016667 0.020833 0.025 0.029167 0.033333 0.0375 0.041667 0.045833 0.05 0.054167 0.058333 0.0625 0.066667 0.070833 0.075 0.079167 0.083333 0.0875 0.091667 0.095833 0.1 0.104167 0.108333 0.1125 0.116667 0.120833 0.125 0.129167 0.133333 0.1375 0.141667 0.15 0.154167 0.158333 0.170833 0.183333 0.1875 0.191667 0.195833 0.2125 0.216667 0.220833 0.225 0.2375 0.241667 0.245833 0.254167 0.258333 0.2625 0.266667 0.283333 0.2875 0.291667 0.295833 0.308333 0.3125 0.316667 0.320833 0.333333 0.3375 0.341667 0.345833 0.358333 0.3625 0.366667 0.375 0.379167 0.383333 0.391667 0.395833 0.4 0.408333 0.4125 0.416667 0.425 0.429167 0.433333 0.441667 0.445833 0.45 0.458333 0.4625 0.466667 0.475 0.479167 0.483333 0.491667 0.495833 0.5 0.508333 0.5125 0.516667 0.525 0.529167 0.533333 0.541667 0.545833 0.55 0.558333 0.5625 0.566667 0.575 0.579167 0.583333 0.591667 0.595833 0.6 0.608333 0.6125 0.616667 0.625 0.629167 0.633333 0.641667 0.645833 0.65 0.658333 0.6625 0.666667 0.675 0.679167 0.683333 0.691667 0.695833 0.7 0.708333 0.7125 0.716667 0.725 0.729167 0.733333 0.741667 0.745833 0.75 0.758333 0.7625 0.766667 0.775 0.779167 0.783333 0.791667 0.795833 0.8 0.804167 0.8125 0.816667 0.820833 0.829167 0.833333 0.8375 0.85 0.854167 0.858333 0.866667 0.870833 0.875 0.879167 0.883333 0.8875 0.891667 0.895833 0.9 0.904167 0.908333 0.9125 0.916667 0.920833 0.925 0.929167 0.933333 0.9375 0.941667 0.945833 0.95 0.954167 0.958333 0.9625 0.966667 0.970833 0.975 0.979167 0.983333 1 1 1 1 1 1
  line L28 (-5.5168, 3.5822) -> (-5.5174, 3.5826)
  line L29 (-4.8225, 3.1314) -> (-5.5168, 3.5822)
  arc A16 (-4.126, 4.0048) -> (-4.8225, 3.1314) centre (0, 0) ccw
  line L30 (-5.455, -1.818) -> (-6.2404, -2.0798)
  line L31 (-6.2404, -2.0798) -> (-6.241, -2.08)
  spline S16 degree 5 poles (-6.241, -2.08) (-6.2411, -2.08) (-6.2412, -2.08) (-6.2415, -2.0801) (-6.2418, -2.0802) (-6.2423, -2.0804) (-6.2429, -2.0806) (-6.2436, -2.0809) (-6.2443, -2.0812) (-6.2451, -2.0815) (-6.246, -2.0818) (-6.247, -2.0822) (-6.248, -2.0826) (-6.2491, -2.083) (-6.2503, -2.0835) (-6.2515, -2.084) (-6.2529, -2.0845) (-6.2542, -2.0851) (-6.2557, -2.0856) (-6.2572, -2.0863) (-6.2587, -2.0869) (-6.2604, -2.0876) (-6.2621, -2.0884) (-6.2638, -2.0891) (-6.2657, -2.0899) (-6.2675, -2.0907) (-6.2695, -2.0916) (-6.2715, -2.0925) (-6.2736, -2.0934) (-6.2757, -2.0944) (-6.2778, -2.0954) (-6.2801, -2.0964) (-6.2824, -2.0975) (-6.2847, -2.0986) (-6.2871, -2.0997) (-6.29, -2.1012) (-6.2931, -2.1026) (-6.2962, -2.1041) (-6.3004, -2.1062) (-6.3059, -2.109) (-6.311, -2.1116) (-6.3162, -2.1143) (-6.3217, -2.1172) (-6.3279, -2.1205) (-6.333, -2.1232) (-6.3382, -2.1261) (-6.3435, -2.129) (-6.3503, -2.1328) (-6.3551, -2.1356) (-6.3601, -2.1384) (-6.3651, -2.1413) (-6.3724, -2.1456) (-6.3783, -2.1491) (-6.3844, -2.1528) (-6.3905, -2.1565) (-6.3984, -2.1613) (-6.4039, -2.1648) (-6.4095, -2.1683) (-6.4152, -2.1719) (-6.4226, -2.1767) (-6.4285, -2.1805) (-6.4344, -2.1843) (-6.4404, -2.1883) (-6.449, -2.194) (-6.456, -2.1987) (-6.4631, -2.2035) (-6.4702, -2.2085) (-6.4792, -2.2148) (-6.4856, -2.2192) (-6.4921, -2.2238) (-6.4986, -2.2285) (-6.507, -2.2346) (-6.5136, -2.2394) (-6.5203, -2.2443) (-6.527, -2.2493) (-6.5357, -2.2558) (-6.5426, -2.261) (-6.5494, -2.2662) (-6.5573, -2.2723) (-6.5653, -2.2785) (-6.5713, -2.2832) (-6.5774, -2.288) (-6.5855, -2.2944) (-6.5926, -2.3001) (-6.5998, -2.3059) (-6.608, -2.3126) (-6.6163, -2.3195) (-6.6226, -2.3246) (-6.6299, -2.3308) (-6.6373, -2.337) (-6.6436, -2.3423) (-6.651, -2.3487) (-6.6585, -2.3551) (-6.6649, -2.3607) (-6.6724, -2.3672) (-6.68, -2.3739) (-6.6865, -2.3797) (-6.6941, -2.3864) (-6.7017, -2.3933) (-6.7083, -2.3993) (-6.716, -2.4063) (-6.7237, -2.4134) (-6.7304, -2.4195) (-6.7381, -2.4268) (-6.7459, -2.4341) (-6.7526, -2.4404) (-6.7604, -2.4479) (-6.7683, -2.4554) (-6.775, -2.4619) (-6.7829, -2.4696) (-6.7908, -2.4774) (-6.7977, -2.4841) (-6.8056, -2.492) (-6.8136, -2.5) (-6.8204, -2.5069) (-6.8284, -2.515) (-6.8364, -2.5232) (-6.8433, -2.5303) (-6.8514, -2.5387) (-6.8595, -2.5471) (-6.8664, -2.5544) (-6.8745, -2.5629) (-6.8826, -2.5716) (-6.8895, -2.5791) (-6.8977, -2.5878) (-6.9058, -2.5967) (-6.9128, -2.6044) (-6.921, -2.6134) (-6.9291, -2.6225) (-6.9362, -2.6303) (-6.9443, -2.6395) (-6.9525, -2.6488) (-6.9596, -2.6569) (-6.9678, -2.6663) (-6.976, -2.6758) (-6.983, -2.684) (-6.9925, -2.6951) (-7.0019, -2.7062) (-7.0101, -2.7161) (-7.0195, -2.7274) (-7.029, -2.7388) (-7.036, -2.7475) (-7.0443, -2.7576) (-7.0525, -2.7678) (-7.0596, -2.7766) (-7.0679, -2.787) (-7.0761, -2.7974) (-7.0832, -2.8064) (-7.0903, -2.8155) (-7.0985, -2.8261) (-7.1056, -2.8353) (-7.1127, -2.8445) (-7.1197, -2.8538) (-7.1268, -2.8632) (-7.1339, -2.8726) (-7.1409, -2.882) (-7.1492, -2.8931) (-7.1574, -2.9042) (-7.1656, -2.9155) (-7.1727, -2.9252) (-7.1797, -2.9349) (-7.1856, -2.9431) (-7.1914, -2.9513) (-7.1973, -2.9595) (-7.2031, -2.9678) (-7.209, -2.9761) (-7.2148, -2.9844) (-7.2207, -2.9928) (-7.2265, -3.0012) (-7.2323, -3.0097) (-7.2381, -3.0182) (-7.244, -3.0267) (-7.2498, -3.0353) (-7.2556, -3.0439) (-7.2614, -3.0525) (-7.2672, -3.0612) (-7.273, -3.0699) (-7.2788, -3.0787) (-7.2846, -3.0875) (-7.2903, -3.0963) (-7.2961, -3.1051) (-7.3019, -3.114) (-7.3076, -3.123) (-7.3168, -3.1373) (-7.3248, -3.15) (-7.3317, -3.1609) (-7.3374, -3.17) (-7.342, -3.1773) knots 0 0 0 0 0 0 0.004167 0.008333 0.0125 0.016667 0.020833 0.025 0.029167 0.033333 0.0375 0.041667 0.045833 0.05 0.054167 0.058333 0.0625 0.066667 0.070833 0.075 0.079167 0.083333 0.0875 0.091667 0.095833 0.1 0.104167 0.108333 0.1125 0.116667 0.120833 0.125 0.129167 0.133333 0.1375 0.141667 0.15 0.154167 0.158333 0.170833 0.183333 0.1875 0.191667 0.195833 0.2125 0.216667 0.220833 0.225 0.2375 0.241667 0.245833 0.25 0.266667 0.270833 0.275 0.279167 0.291667 0.295833 0.3 0.304167 0.316667 0.320833 0.325 0.329167 0.345833 0.35 0.354167 0.358333 0.370833 0.375 0.379167 0.383333 0.395833 0.4 0.404167 0.408333 0.420833 0.425 0.429167 0.4375 0.441667 0.445833 0.45 0.4625 0.466667 0.470833 0.479167 0.483333 0.4875 0.495833 0.5 0.504167 0.5125 0.516667 0.520833 0.529167 0.533333 0.5375 0.545833 0.55 0.554167 0.5625 0.566667 0.570833 0.579167 0.583333 0.5875 0.595833 0.6 0.604167 0.6125 0.616667 0.620833 0.629167 0.633333 0.6375 0.645833 0.65 0.654167 0.6625 0.666667 0.670833 0.679167 0.683333 0.6875 0.695833 0.7 0.704167 0.7125 0.716667 0.720833 0.729167 0.733333 0.7375 0.745833 0.75 0.754167 0.766667 0.770833 0.775 0.783333 0.7875 0.791667 0.8 0.804167 0.808333 0.816667 0.820833 0.825 0.829167 0.8375 0.841667 0.845833 0.85 0.854167 0.8625 0.866667 0.875 0.879167 0.883333 0.8875 0.891667 0.895833 0.9 0.904167 0.908333 0.9125 0.916667 0.920833 0.925 0.929167 0.933333 0.9375 0.941667 0.945833 0.95 0.954167 0.958333 0.9625 0.966667 0.970833 0.975 0.979167 0.983333 1 1 1 1 1 1
  arc A17 (-7.342, -3.1773) -> (-7.0618, -3.7592) centre (0, 0) ccw
  spline S17 degree 5 poles (-7.0618, -3.7592) (-7.0553, -3.7599) (-7.0468, -3.7609) (-7.0361, -3.7621) (-7.0233, -3.7635) (-7.0084, -3.7651) (-6.9979, -3.7662) (-6.9873, -3.7673) (-6.9767, -3.7683) (-6.9662, -3.7693) (-6.9557, -3.7703) (-6.9452, -3.7713) (-6.9348, -3.7722) (-6.9244, -3.7731) (-6.914, -3.774) (-6.9036, -3.7748) (-6.8933, -3.7756) (-6.8829, -3.7764) (-6.8726, -3.7772) (-6.8624, -3.7779) (-6.8521, -3.7787) (-6.8419, -3.7793) (-6.8317, -3.78) (-6.8215, -3.7806) (-6.8114, -3.7812) (-6.8013, -3.7818) (-6.7912, -3.7824) (-6.7811, -3.7829) (-6.7711, -3.7834) (-6.7611, -3.7839) (-6.7511, -3.7843) (-6.7372, -3.7849) (-6.7233, -3.7855) (-6.7095, -3.786) (-6.6957, -3.7864) (-6.6781, -3.7869) (-6.6605, -3.7873) (-6.6431, -3.7877) (-6.6258, -3.7879) (-6.6085, -3.7881) (-6.5914, -3.7882) (-6.5781, -3.7882) (-6.5649, -3.7882) (-6.5518, -3.7881) (-6.5331, -3.788) (-6.5182, -3.7878) (-6.5034, -3.7875) (-6.4887, -3.7872) (-6.4705, -3.7867) (-6.4578, -3.7863) (-6.4451, -3.7858) (-6.4325, -3.7854) (-6.4164, -3.7847) (-6.404, -3.7841) (-6.3916, -3.7835) (-6.3793, -3.7828) (-6.3618, -3.7818) (-6.3479, -3.781) (-6.3342, -3.7801) (-6.3205, -3.7791) (-6.3035, -3.7778) (-6.2916, -3.7769) (-6.2799, -3.7759) (-6.2682, -3.7749) (-6.2533, -3.7735) (-6.2417, -3.7724) (-6.2303, -3.7713) (-6.2173, -3.7699) (-6.2044, -3.7685) (-6.1947, -3.7675) (-6.1836, -3.7662) (-6.1725, -3.7649) (-6.1631, -3.7637) (-6.1521, -3.7623) (-6.1412, -3.7609) (-6.132, -3.7597) (-6.1212, -3.7582) (-6.1106, -3.7568) (-6.1015, -3.7555) (-6.091, -3.7539) (-6.0805, -3.7523) (-6.0716, -3.751) (-6.0613, -3.7493) (-6.0511, -3.7477) (-6.0424, -3.7462) (-6.0323, -3.7445) (-6.0223, -3.7428) (-6.0138, -3.7413) (-6.004, -3.7395) (-5.9942, -3.7377) (-5.9859, -3.7361) (-5.9763, -3.7343) (-5.9667, -3.7324) (-5.9586, -3.7308) (-5.9493, -3.7289) (-5.94, -3.727) (-5.9321, -3.7253) (-5.9229, -3.7233) (-5.9139, -3.7214) (-5.9062, -3.7196) (-5.8973, -3.7176) (-5.8885, -3.7156) (-5.881, -3.7138) (-5.8723, -3.7118) (-5.8638, -3.7097) (-5.8565, -3.7079) (-5.8481, -3.7058) (-5.8398, -3.7037) (-5.8328, -3.7019) (-5.8246, -3.6997) (-5.8166, -3.6976) (-5.8098, -3.6957) (-5.8019, -3.6935) (-5.7941, -3.6914) (-5.7875, -3.6895) (-5.7799, -3.6873) (-5.7724, -3.6851) (-5.766, -3.6832) (-5.7587, -3.681) (-5.7514, -3.6788) (-5.7453, -3.6769) (-5.7382, -3.6747) (-5.7313, -3.6725) (-5.7254, -3.6706) (-5.7186, -3.6684) (-5.7119, -3.6662) (-5.7063, -3.6643) (-5.6998, -3.6621) (-5.6934, -3.6599) (-5.688, -3.658) (-5.6817, -3.6558) (-5.6756, -3.6536) (-5.6705, -3.6518) (-5.6646, -3.6496) (-5.6588, -3.6474) (-5.6539, -3.6456) (-5.6483, -3.6435) (-5.6428, -3.6413) (-5.6381, -3.6395) (-5.6328, -3.6374) (-5.6276, -3.6353) (-5.6232, -3.6336) (-5.6182, -3.6315) (-5.6133, -3.6295) (-5.6079, -3.6272) (-5.6026, -3.625) (-5.5974, -3.6227) (-5.593, -3.6208) (-5.5876, -3.6184) (-5.5834, -3.6165) (-5.5794, -3.6147) (-5.5755, -3.6129) (-5.5717, -3.6111) (-5.5691, -3.6099) (-5.5665, -3.6087) (-5.564, -3.6075) (-5.5616, -3.6063) (-5.5592, -3.6051) (-5.5569, -3.604) (-5.5546, -3.6029) (-5.5524, -3.6018) (-5.5503, -3.6007) (-5.5482, -3.5996) (-5.5462, -3.5986) (-5.5442, -3.5976) (-5.5424, -3.5966) (-5.5405, -3.5957) (-5.5388, -3.5947) (-5.5371, -3.5938) (-5.5355, -3.593) (-5.5339, -3.5921) (-5.5324, -3.5913) (-5.531, -3.5905) (-5.5296, -3.5897) (-5.5283, -3.589) (-5.5271, -3.5883) (-5.5259, -3.5877) (-5.5248, -3.587) (-5.5238, -3.5864) (-5.5228, -3.5859) (-5.522, -3.5854) (-5.5211, -3.5849) (-5.5204, -3.5844) (-5.5197, -3.584) (-5.5191, -3.5837) (-5.5185, -3.5833) (-5.518, -3.583) (-5.5177, -3.5828) (-5.5175, -3.5827) (-5.5174, -3.5826) knots -1 -1 -1 -1 -1 -1 -0.9875 -0.983333 -0.979167 -0.975 -0.970833 -0.966667 -0.9625 -0.958333 -0.954167 -0.95 -0.945833 -0.941667 -0.9375 -0.933333 -0.929167 -0.925 -0.920833 -0.916667 -0.9125 -0.908333 -0.904167 -0.9 -0.895833 -0.891667 -0.8875 -0.883333 -0.879167 -0.875 -0.870833 -0.866667 -0.854167 -0.85 -0.845833 -0.841667 -0.829167 -0.816667 -0.8125 -0.808333 -0.804167 -0.791667 -0.7875 -0.783333 -0.779167 -0.7625 -0.758333 -0.754167 -0.75 -0.7375 -0.733333 -0.729167 -0.725 -0.7125 -0.708333 -0.704167 -0.7 -0.683333 -0.679167 -0.675 -0.670833 -0.658333 -0.654167 -0.65 -0.645833 -0.633333 -0.629167 -0.625 -0.616667 -0.6125 -0.608333 -0.6 -0.595833 -0.591667 -0.583333 -0.579167 -0.575 -0.566667 -0.5625 -0.558333 -0.55 -0.545833 -0.541667 -0.533333 -0.529167 -0.525 -0.516667 -0.5125 -0.508333 -0.5 -0.495833 -0.491667 -0.483333 -0.479167 -0.475 -0.466667 -0.4625 -0.458333 -0.45 -0.445833 -0.441667 -0.433333 -0.429167 -0.425 -0.416667 -0.4125 -0.408333 -0.4 -0.395833 -0.391667 -0.383333 -0.379167 -0.375 -0.366667 -0.3625 -0.358333 -0.35 -0.345833 -0.341667 -0.333333 -0.329167 -0.325 -0.316667 -0.3125 -0.308333 -0.3 -0.295833 -0.291667 -0.283333 -0.279167 -0.275 -0.266667 -0.2625 -0.258333 -0.25 -0.245833 -0.241667 -0.233333 -0.229167 -0.225 -0.216667 -0.2125 -0.208333 -0.2 -0.195833 -0.183333 -0.179167 -0.175 -0.170833 -0.158333 -0.154167 -0.15 -0.145833 -0.141667 -0.1375 -0.133333 -0.129167 -0.125 -0.120833 -0.116667 -0.1125 -0.108333 -0.104167 -0.1 -0.095833 -0.091667 -0.0875 -0.083333 -0.079167 -0.075 -0.070833 -0.066667 -0.0625 -0.058333 -0.054167 -0.05 -0.045833 -0.041667 -0.0375 -0.033333 -0.029167 -0.025 -0.020833 -0.016667 -0.0125 -0.008333 0 0 0 0 0 0
  line L32 (-5.5168, -3.5822) -> (-4.8225, -3.1314)
  line L33 (-5.5174, -3.5826) -> (-5.5168, -3.5822)
  arc A18 (-4.8225, -3.1314) -> (-4.126, -4.0048) centre (0, 0) ccw
  line L34 (-4.126, -4.0048) -> (-4.72, -4.5814)
  line L35 (-4.72, -4.5814) -> (-4.7205, -4.5819)
  line L36 (-3.4162, -5.6212) -> (-2.9863, -4.9137)